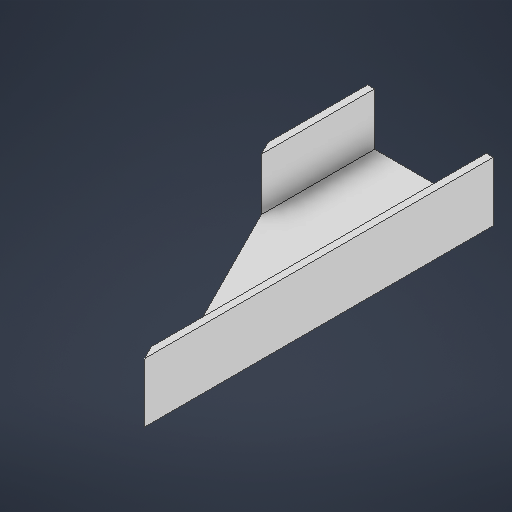
# Autodesk Inventor part: outside2
Saved by Autodesk Inventor 2026.2 (Build 302298000, 298)
## iProperties
Created: 2026-03-14
Part Number: outside2
Material: Generic
Document SubType Name: Modeling
Designer: danda
Density: 1 g/cm^3
Appearance: Default
Author: danda
Autodesk Inventor part; units mm, degrees
ref_plane "YZ Plane" through (0, 0, 0) normal (1, 0, 0) x (0, 1, 0)
ref_plane "XZ Plane" through (0, 0, 0) normal (0, 1, 0) x (-1, 0, 0)
ref_plane "XY Plane" through (0, 0, 0) normal (0, 0, 1) x (1, 0, 0)
sketch "Sketch1" plane through (0, 0, 0) normal (0, 0, 1) x (1, 0, 0)
  line L0 (13.3295, 18.9186) -> (13.3295, 3.9186)
  line L1 (13.3295, 3.9186) -> (45.3295, 3.9186)
  line L2 (45.3295, 3.9186) -> (45.3295, 18.9186)
  line L3 (11.3295, 18.9186) -> (11.3295, 1.9186)
  line L4 (11.3295, 1.9186) -> (47.3295, 1.9186)
  line L5 (47.3295, 1.9186) -> (47.3295, 18.9186)
  line L6 (13.3295, 18.9186) -> (11.3295, 18.9186)
  line L7 (45.3295, 18.9186) -> (47.3295, 18.9186)
  point P0 (0, 0)
  dimension "d0" = 15
  dimension "d1" = 32
  dimension "d2" = 2
  constraints: 16 end point, 4 perpendicular, 1 collinear, 1 horizontal, 1 vertical, 2 other
  measures "d0" distance of L0.start L0.end
  measures "d1" distance of L0.end L1.end
  measures "d2" distance between parallel lines of L0 L3
extrude "Extrusion1" add sketch "Sketch1" along normal blind 100
sketch "Sketch2" plane through (13.3295, 3.9186, 0) normal (0, 1, 0) x (1, 0, 0)
  line L0 (34, -100) -> (32, -100) projected
  line L1 (34, -100) -> (-2.138, -28.2724)
  line L2 (34, -100) -> (114.3169, -100) construction
  line L3 (32, -100) -> (0, -100) projected
  line L4 (34, -100) -> (-2.138, -100)
  line L5 (-2.138, -100) -> (-2.138, -28.2724)
  point P0 (-13.3295, 0)
  point P1 (0, -100)
  dimension "d5" = 116.74
  dimension "d6" = 63.26
  constraints: 8 end point, 1 equal length, 1 horizontal, 1 perpendicular, 1 point on line
  measures "d5" angle of L2 L1
  measures "d6" angle of L3 L1
extrude "Extrusion2" cut sketch "Sketch2" along normal through all both and the other way through all
body "Solid1"
